Autodesk Inventor part; units mm, degrees
(part 2 of 3)
sketch "Эскиз3" plane through (0, 10, 0) normal (0, 1, 0) x (1, 0, 0)
  line L0 (-500, 500) -> (-500, -500) projected
  line L1 (-500, -500) -> (500, -500) projected
  line L2 (500, -500) -> (500, 500) projected
  line L3 (500, 500) -> (-500, 500) projected
  line L4 (-97.5, 500) -> (-102.5, 500) projected
  line L5 (-102.5, 500) -> (-102.5, 402.5) projected
  line L6 (-102.5, 402.5) -> (-197.5, 402.5) projected
  line L7 (-197.5, 402.5) -> (-197.5, 500) projected
  line L8 (-197.5, 500) -> (-202.5, 500) projected
  line L9 (-202.5, 500) -> (-202.5, 402.5) projected
  line L10 (-202.5, 402.5) -> (-297.5, 402.5) projected
  line L11 (-297.5, 402.5) -> (-297.5, 500) projected
  line L12 (-297.5, 500) -> (-302.5, 500) projected
  line L13 (-302.5, 500) -> (-302.5, 402.5) projected
  line L14 (-302.5, 402.5) -> (-397.5, 402.5) projected
  line L15 (-397.5, 402.5) -> (-397.5, 500) projected
  line L16 (-397.5, 500) -> (-402.5, 500) projected
  line L17 (-402.5, 500) -> (-402.5, 402.5) projected
  line L18 (-402.5, 402.5) -> (-500, 402.5) projected
  line L19 (-500, 402.5) -> (-500, 397.5) projected
  line L20 (-500, 397.5) -> (-402.5, 397.5) projected
  line L21 (-402.5, 397.5) -> (-402.5, 302.5) projected
  line L22 (-402.5, 302.5) -> (-500, 302.5) projected
  line L23 (-500, 302.5) -> (-500, 297.5) projected
  line L24 (-500, 297.5) -> (-402.5, 297.5) projected
  line L25 (-402.5, 297.5) -> (-402.5, 202.5) projected
  line L26 (-402.5, 202.5) -> (-500, 202.5) projected
  line L27 (-500, 202.5) -> (-500, 197.5) projected
  line L28 (-500, 197.5) -> (-402.5, 197.5) projected
  line L29 (-402.5, 197.5) -> (-402.5, 102.5) projected
  line L30 (-402.5, 102.5) -> (-500, 102.5) projected
  line L31 (-500, 102.5) -> (-500, 97.5) projected
  line L32 (-500, 97.5) -> (-402.5, 97.5) projected
  line L33 (-402.5, 97.5) -> (-402.5, 2.5) projected
  line L34 (-402.5, 2.5) -> (-500, 2.5) projected
  line L35 (-500, 2.5) -> (-500, -2.5) projected
  line L36 (-500, -2.5) -> (-402.5, -2.5) projected
  line L37 (-402.5, -2.5) -> (-402.5, -97.5) projected
  line L38 (-402.5, -97.5) -> (-500, -97.5) projected
  line L39 (-500, -97.5) -> (-500, -102.5) projected
  line L40 (-500, -102.5) -> (-402.5, -102.5) projected
  line L41 (-402.5, -102.5) -> (-402.5, -197.5) projected
  line L42 (-402.5, -197.5) -> (-500, -197.5) projected
  line L43 (-500, -197.5) -> (-500, -202.5) projected
  line L44 (-500, -202.5) -> (-402.5, -202.5) projected
  line L45 (-402.5, -202.5) -> (-402.5, -297.5) projected
  line L46 (-402.5, -297.5) -> (-500, -297.5) projected
  line L47 (-500, -297.5) -> (-500, -302.5) projected
  line L48 (-500, -302.5) -> (-402.5, -302.5) projected
  line L49 (-402.5, -302.5) -> (-402.5, -397.5) projected
  line L50 (-402.5, -397.5) -> (-500, -397.5) projected
  line L51 (-500, -397.5) -> (-500, -402.5) projected
  line L52 (-500, -402.5) -> (-402.5, -402.5) projected
  line L53 (-402.5, -402.5) -> (-402.5, -500) projected
  line L54 (-402.5, -500) -> (-397.5, -500) projected
  line L55 (-397.5, -500) -> (-397.5, -402.5) projected
  line L56 (-397.5, -402.5) -> (-302.5, -402.5) projected
  line L57 (-302.5, -402.5) -> (-302.5, -500) projected
  line L58 (-302.5, -500) -> (-297.5, -500) projected
  line L59 (-297.5, -500) -> (-297.5, -402.5) projected
  line L60 (-297.5, -402.5) -> (-202.5, -402.5) projected
  line L61 (-202.5, -402.5) -> (-202.5, -500) projected
  line L62 (-202.5, -500) -> (-197.5, -500) projected
  line L63 (-197.5, -500) -> (-197.5, -402.5) projected
  line L64 (-197.5, -402.5) -> (-102.5, -402.5) projected
  line L65 (-102.5, -402.5) -> (-102.5, -500) projected
  line L66 (-102.5, -500) -> (-97.5, -500) projected
  line L67 (-97.5, -500) -> (-97.5, -402.5) projected
  line L68 (-97.5, -402.5) -> (-2.5, -402.5) projected
  line L69 (-2.5, -402.5) -> (-2.5, -500) projected
  line L70 (-2.5, -500) -> (2.5, -500) projected
  line L71 (2.5, -500) -> (2.5, -402.5) projected
  line L72 (2.5, -402.5) -> (97.5, -402.5) projected
  line L73 (97.5, -402.5) -> (97.5, -500) projected
  line L74 (97.5, -500) -> (102.5, -500) projected
  line L75 (102.5, -500) -> (102.5, -402.5) projected
  line L76 (102.5, -402.5) -> (197.5, -402.5) projected
  line L77 (197.5, -402.5) -> (197.5, -500) projected
  line L78 (197.5, -500) -> (202.5, -500) projected
  line L79 (202.5, -500) -> (202.5, -402.5) projected
  line L80 (202.5, -402.5) -> (297.5, -402.5) projected
  line L81 (297.5, -402.5) -> (297.5, -500) projected
  line L82 (297.5, -500) -> (302.5, -500) projected
  line L83 (302.5, -500) -> (302.5, -402.5) projected
  line L84 (302.5, -402.5) -> (397.5, -402.5) projected
  line L85 (397.5, -402.5) -> (397.5, -500) projected
  line L86 (397.5, -500) -> (402.5, -500) projected
  line L87 (402.5, -500) -> (402.5, -402.5) projected
  line L88 (402.5, -402.5) -> (500, -402.5) projected
  line L89 (500, -402.5) -> (500, -397.5) projected
  line L90 (500, -397.5) -> (402.5, -397.5) projected
  line L91 (402.5, -397.5) -> (402.5, -302.5) projected
  line L92 (402.5, -302.5) -> (500, -302.5) projected
  line L93 (500, -302.5) -> (500, -297.5) projected
  line L94 (500, -297.5) -> (402.5, -297.5) projected
  line L95 (402.5, -297.5) -> (402.5, -202.5) projected
  line L96 (402.5, -202.5) -> (500, -202.5) projected
  line L97 (500, -202.5) -> (500, -197.5) projected
  line L98 (500, -197.5) -> (402.5, -197.5) projected
  line L99 (402.5, -197.5) -> (402.5, -102.5) projected
  line L100 (402.5, -102.5) -> (500, -102.5) projected
  line L101 (500, -102.5) -> (500, -97.5) projected
  line L102 (500, -97.5) -> (402.5, -97.5) projected
  line L103 (402.5, -97.5) -> (402.5, -2.5) projected
  line L104 (402.5, -2.5) -> (500, -2.5) projected
  line L105 (500, -2.5) -> (500, 2.5) projected
  line L106 (500, 2.5) -> (402.5, 2.5) projected
  line L107 (402.5, 2.5) -> (402.5, 97.5) projected
  line L108 (402.5, 97.5) -> (500, 97.5) projected
  line L109 (500, 97.5) -> (500, 102.5) projected
  line L110 (500, 102.5) -> (402.5, 102.5) projected
  line L111 (402.5, 102.5) -> (402.5, 197.5) projected
  line L112 (402.5, 197.5) -> (500, 197.5) projected
  line L113 (500, 197.5) -> (500, 202.5) projected
  line L114 (500, 202.5) -> (402.5, 202.5) projected
  line L115 (402.5, 202.5) -> (402.5, 297.5) projected
  line L116 (402.5, 297.5) -> (500, 297.5) projected
  line L117 (500, 297.5) -> (500, 302.5) projected
  line L118 (500, 302.5) -> (402.5, 302.5) projected
  line L119 (402.5, 302.5) -> (402.5, 397.5) projected
  line L120 (402.5, 397.5) -> (500, 397.5) projected
  line L121 (500, 397.5) -> (500, 402.5) projected
  line L122 (500, 402.5) -> (402.5, 402.5) projected
  line L123 (402.5, 402.5) -> (402.5, 500) projected
  line L124 (402.5, 500) -> (397.5, 500) projected
  line L125 (397.5, 500) -> (397.5, 402.5) projected
  line L126 (397.5, 402.5) -> (302.5, 402.5) projected
  line L127 (302.5, 402.5) -> (302.5, 500) projected
  line L128 (302.5, 500) -> (297.5, 500) projected
  line L129 (297.5, 500) -> (297.5, 402.5) projected
  line L130 (297.5, 402.5) -> (202.5, 402.5) projected
  line L131 (202.5, 402.5) -> (202.5, 500) projected
  line L132 (202.5, 500) -> (197.5, 500) projected
  line L133 (197.5, 500) -> (197.5, 402.5) projected
  line L134 (197.5, 402.5) -> (102.5, 402.5) projected
  line L135 (102.5, 402.5) -> (102.5, 500) projected
  line L136 (102.5, 500) -> (97.5, 500) projected
  line L137 (97.5, 500) -> (97.5, 402.5) projected
  line L138 (97.5, 402.5) -> (2.5, 402.5) projected
  line L139 (2.5, 402.5) -> (2.5, 500) projected
  line L140 (2.5, 500) -> (-2.5, 500) projected
  line L141 (-2.5, 500) -> (-2.5, 402.5) projected
  line L142 (-2.5, 402.5) -> (-97.5, 402.5) projected
  line L143 (-97.5, 402.5) -> (-97.5, 500) projected
  line L144 (197.5, -302.5) -> (197.5, -397.5) projected
  line L145 (197.5, -397.5) -> (102.5, -397.5) projected
  line L146 (102.5, -397.5) -> (102.5, -302.5) projected
  line L147 (102.5, -302.5) -> (197.5, -302.5) projected
  line L148 (197.5, -297.5) -> (102.5, -297.5) projected
  line L149 (102.5, -297.5) -> (102.5, -202.5) projected
  line L150 (102.5, -202.5) -> (197.5, -202.5) projected
  line L151 (197.5, -202.5) -> (197.5, -297.5) projected
  line L152 (97.5, -102.5) -> (97.5, -197.5) projected
  line L153 (97.5, -197.5) -> (2.5, -197.5) projected
  line L154 (2.5, -197.5) -> (2.5, -102.5) projected
  line L155 (2.5, -102.5) -> (97.5, -102.5) projected
  line L156 (97.5, -97.5) -> (2.5, -97.5) projected
  line L157 (2.5, -97.5) -> (2.5, -2.5) projected
  line L158 (2.5, -2.5) -> (97.5, -2.5) projected
  line L159 (97.5, -2.5) -> (97.5, -97.5) projected
  line L160 (-2.5, 97.5) -> (-2.5, 2.5) projected
  line L161 (-2.5, 2.5) -> (-97.5, 2.5) projected
  line L162 (-97.5, 2.5) -> (-97.5, 97.5) projected
  line L163 (-97.5, 97.5) -> (-2.5, 97.5) projected
  line L164 (-2.5, 102.5) -> (-97.5, 102.5) projected
  line L165 (-97.5, 102.5) -> (-97.5, 197.5) projected
  line L166 (-97.5, 197.5) -> (-2.5, 197.5) projected
  line L167 (-2.5, 197.5) -> (-2.5, 102.5) projected
  line L168 (-97.5, 397.5) -> (-2.5, 397.5) projected
  line L169 (-2.5, 397.5) -> (-2.5, 302.5) projected
  line L170 (-2.5, 302.5) -> (-97.5, 302.5) projected
  line L171 (-97.5, 302.5) -> (-97.5, 397.5) projected
  line L172 (-97.5, 297.5) -> (-2.5, 297.5) projected
  line L173 (-2.5, 297.5) -> (-2.5, 202.5) projected
  line L174 (-2.5, 202.5) -> (-97.5, 202.5) projected
  line L175 (-97.5, 202.5) -> (-97.5, 297.5) projected
  line L176 (-102.5, -302.5) -> (-102.5, -397.5) projected
  line L177 (-102.5, -397.5) -> (-197.5, -397.5) projected
  line L178 (-197.5, -397.5) -> (-197.5, -302.5) projected
  line L179 (-197.5, -302.5) -> (-102.5, -302.5) projected
  line L180 (-102.5, -202.5) -> (-102.5, -297.5) projected
  line L181 (-102.5, -297.5) -> (-197.5, -297.5) projected
  line L182 (-197.5, -297.5) -> (-197.5, -202.5) projected
  line L183 (-197.5, -202.5) -> (-102.5, -202.5) projected
  line L184 (-102.5, -102.5) -> (-102.5, -197.5) projected
  line L185 (-102.5, -197.5) -> (-197.5, -197.5) projected
  line L186 (-197.5, -197.5) -> (-197.5, -102.5) projected
  line L187 (-197.5, -102.5) -> (-102.5, -102.5) projected
  line L188 (-102.5, -2.5) -> (-102.5, -97.5) projected
  line L189 (-102.5, -97.5) -> (-197.5, -97.5) projected
  line L190 (-197.5, -97.5) -> (-197.5, -2.5) projected
  line L191 (-197.5, -2.5) -> (-102.5, -2.5) projected
  line L192 (-102.5, 97.5) -> (-102.5, 2.5) projected
  line L193 (-102.5, 2.5) -> (-197.5, 2.5) projected
  line L194 (-197.5, 2.5) -> (-197.5, 97.5) projected
  line L195 (-197.5, 97.5) -> (-102.5, 97.5) projected
  line L196 (-102.5, 197.5) -> (-102.5, 102.5) projected
  line L197 (-102.5, 102.5) -> (-197.5, 102.5) projected
  line L198 (-197.5, 102.5) -> (-197.5, 197.5) projected
  line L199 (-197.5, 197.5) -> (-102.5, 197.5) projected
  line L200 (-102.5, 297.5) -> (-102.5, 202.5) projected
  line L201 (-102.5, 202.5) -> (-197.5, 202.5) projected
  line L202 (-197.5, 202.5) -> (-197.5, 297.5) projected
  line L203 (-197.5, 297.5) -> (-102.5, 297.5) projected
  line L204 (-102.5, 397.5) -> (-102.5, 302.5) projected
  line L205 (-102.5, 302.5) -> (-197.5, 302.5) projected
  line L206 (-197.5, 302.5) -> (-197.5, 397.5) projected
  line L207 (-197.5, 397.5) -> (-102.5, 397.5) projected
  line L208 (-97.5, -302.5) -> (-2.5, -302.5) projected
  line L209 (-2.5, -302.5) -> (-2.5, -397.5) projected
  line L210 (-2.5, -397.5) -> (-97.5, -397.5) projected
  line L211 (-97.5, -397.5) -> (-97.5, -302.5) projected
  line L212 (-202.5, -302.5) -> (-202.5, -397.5) projected
  line L213 (-202.5, -397.5) -> (-297.5, -397.5) projected
  line L214 (-297.5, -397.5) -> (-297.5, -302.5) projected
  line L215 (-297.5, -302.5) -> (-202.5, -302.5) projected
  line L216 (-202.5, -297.5) -> (-297.5, -297.5) projected
  line L217 (-297.5, -297.5) -> (-297.5, -202.5) projected
  line L218 (-297.5, -202.5) -> (-202.5, -202.5) projected
  line L219 (-202.5, -202.5) -> (-202.5, -297.5) projected
  line L220 (2.5, 102.5) -> (2.5, 197.5) projected
  line L221 (2.5, 197.5) -> (97.5, 197.5) projected
  line L222 (97.5, 197.5) -> (97.5, 102.5) projected
  line L223 (97.5, 102.5) -> (2.5, 102.5) projected
  line L224 (-297.5, 397.5) -> (-202.5, 397.5) projected
  line L225 (-202.5, 397.5) -> (-202.5, 302.5) projected
  line L226 (-202.5, 302.5) -> (-297.5, 302.5) projected
  line L227 (-297.5, 302.5) -> (-297.5, 397.5) projected
  line L228 (-297.5, 297.5) -> (-202.5, 297.5) projected
  line L229 (-202.5, 297.5) -> (-202.5, 202.5) projected
  line L230 (-202.5, 202.5) -> (-297.5, 202.5) projected
  line L231 (-297.5, 202.5) -> (-297.5, 297.5) projected
  line L232 (-297.5, 197.5) -> (-202.5, 197.5) projected
  line L233 (-202.5, 197.5) -> (-202.5, 102.5) projected
  line L234 (-202.5, 102.5) -> (-297.5, 102.5) projected
  line L235 (-297.5, 102.5) -> (-297.5, 197.5) projected
  line L236 (-297.5, 97.5) -> (-202.5, 97.5) projected
  line L237 (-202.5, 97.5) -> (-202.5, 2.5) projected
  line L238 (-202.5, 2.5) -> (-297.5, 2.5) projected
  line L239 (-297.5, 2.5) -> (-297.5, 97.5) projected
  line L240 (-297.5, -2.5) -> (-202.5, -2.5) projected
  line L241 (-202.5, -2.5) -> (-202.5, -97.5) projected
  line L242 (-202.5, -97.5) -> (-297.5, -97.5) projected
  line L243 (-297.5, -97.5) -> (-297.5, -2.5) projected
  line L244 (-297.5, -102.5) -> (-202.5, -102.5) projected
  line L245 (-202.5, -102.5) -> (-202.5, -197.5) projected
  line L246 (-202.5, -197.5) -> (-297.5, -197.5) projected
  line L247 (-297.5, -197.5) -> (-297.5, -102.5) projected
  line L248 (-302.5, -302.5) -> (-302.5, -397.5) projected
  line L249 (-302.5, -397.5) -> (-397.5, -397.5) projected
  line L250 (-397.5, -397.5) -> (-397.5, -302.5) projected
  line L251 (-397.5, -302.5) -> (-302.5, -302.5) projected
  line L252 (-302.5, -202.5) -> (-302.5, -297.5) projected
  line L253 (-302.5, -297.5) -> (-397.5, -297.5) projected
  line L254 (-397.5, -297.5) -> (-397.5, -202.5) projected
  line L255 (-397.5, -202.5) -> (-302.5, -202.5) projected
  line L256 (-302.5, -102.5) -> (-302.5, -197.5) projected
  line L257 (-302.5, -197.5) -> (-397.5, -197.5) projected
  line L258 (-397.5, -197.5) -> (-397.5, -102.5) projected
  line L259 (-397.5, -102.5) -> (-302.5, -102.5) projected
  line L260 (-302.5, -2.5) -> (-302.5, -97.5) projected
  line L261 (-302.5, -97.5) -> (-397.5, -97.5) projected
  line L262 (-397.5, -97.5) -> (-397.5, -2.5) projected
  line L263 (-397.5, -2.5) -> (-302.5, -2.5) projected
  line L264 (-302.5, 97.5) -> (-302.5, 2.5) projected
  line L265 (-302.5, 2.5) -> (-397.5, 2.5) projected
  line L266 (-397.5, 2.5) -> (-397.5, 97.5) projected
  line L267 (-397.5, 97.5) -> (-302.5, 97.5) projected
  line L268 (-302.5, 197.5) -> (-302.5, 102.5) projected
  line L269 (-302.5, 102.5) -> (-397.5, 102.5) projected
  line L270 (-397.5, 102.5) -> (-397.5, 197.5) projected
  line L271 (-397.5, 197.5) -> (-302.5, 197.5) projected
  line L272 (-302.5, 297.5) -> (-302.5, 202.5) projected
  line L273 (-302.5, 202.5) -> (-397.5, 202.5) projected
  line L274 (-397.5, 202.5) -> (-397.5, 297.5) projected
  line L275 (-397.5, 297.5) -> (-302.5, 297.5) projected
  line L276 (-302.5, 397.5) -> (-302.5, 302.5) projected
  line L277 (-302.5, 302.5) -> (-397.5, 302.5) projected
  line L278 (-397.5, 302.5) -> (-397.5, 397.5) projected
  line L279 (-397.5, 397.5) -> (-302.5, 397.5) projected
  line L280 (-97.5, -102.5) -> (-2.5, -102.5) projected
  line L281 (-2.5, -102.5) -> (-2.5, -197.5) projected
  line L282 (-2.5, -197.5) -> (-97.5, -197.5) projected
  line L283 (-97.5, -197.5) -> (-97.5, -102.5) projected
  line L284 (-97.5, -2.5) -> (-2.5, -2.5) projected
  line L285 (-2.5, -2.5) -> (-2.5, -97.5) projected
  line L286 (-2.5, -97.5) -> (-97.5, -97.5) projected
  line L287 (-97.5, -97.5) -> (-97.5, -2.5) projected
  line L288 (2.5, 97.5) -> (97.5, 97.5) projected
  line L289 (97.5, 97.5) -> (97.5, 2.5) projected
  line L290 (97.5, 2.5) -> (2.5, 2.5) projected
  line L291 (2.5, 2.5) -> (2.5, 97.5) projected
  line L292 (202.5, -297.5) -> (202.5, -202.5) projected
  line L293 (202.5, -202.5) -> (297.5, -202.5) projected
  line L294 (297.5, -202.5) -> (297.5, -297.5) projected
  line L295 (297.5, -297.5) -> (202.5, -297.5) projected
  line L296 (102.5, -102.5) -> (197.5, -102.5) projected
  line L297 (197.5, -102.5) -> (197.5, -197.5) projected
  line L298 (197.5, -197.5) -> (102.5, -197.5) projected
  line L299 (102.5, -197.5) -> (102.5, -102.5) projected
  line L300 (202.5, -302.5) -> (297.5, -302.5) projected
  line L301 (297.5, -302.5) -> (297.5, -397.5) projected
  line L302 (297.5, -397.5) -> (202.5, -397.5) projected
  line L303 (202.5, -397.5) -> (202.5, -302.5) projected
  line L304 (202.5, -97.5) -> (202.5, -2.5) projected
  line L305 (202.5, -2.5) -> (297.5, -2.5) projected
  line L306 (297.5, -2.5) -> (297.5, -97.5) projected
  line L307 (297.5, -97.5) -> (202.5, -97.5) projected
  line L308 (197.5, 2.5) -> (102.5, 2.5) projected
  line L309 (102.5, 2.5) -> (102.5, 97.5) projected
  line L310 (102.5, 97.5) -> (197.5, 97.5) projected
  line L311 (197.5, 97.5) -> (197.5, 2.5) projected
  line L312 (202.5, 102.5) -> (202.5, 197.5) projected
  line L313 (202.5, 197.5) -> (297.5, 197.5) projected
  line L314 (297.5, 197.5) -> (297.5, 102.5) projected
  line L315 (297.5, 102.5) -> (202.5, 102.5) projected
  line L316 (197.5, 202.5) -> (102.5, 202.5) projected
  line L317 (102.5, 202.5) -> (102.5, 297.5) projected
  line L318 (102.5, 297.5) -> (197.5, 297.5) projected
  line L319 (197.5, 297.5) -> (197.5, 202.5) projected
  line L320 (202.5, 302.5) -> (202.5, 397.5) projected
  line L321 (202.5, 397.5) -> (297.5, 397.5) projected
  line L322 (297.5, 397.5) -> (297.5, 302.5) projected
  line L323 (297.5, 302.5) -> (202.5, 302.5) projected
  line L324 (97.5, -202.5) -> (97.5, -297.5) projected
  line L325 (97.5, -297.5) -> (2.5, -297.5) projected
  line L326 (2.5, -297.5) -> (2.5, -202.5) projected
  line L327 (2.5, -202.5) -> (97.5, -202.5) projected
  line L328 (97.5, -302.5) -> (97.5, -397.5) projected
  line L329 (97.5, -397.5) -> (2.5, -397.5) projected
  line L330 (2.5, -397.5) -> (2.5, -302.5) projected
  line L331 (2.5, -302.5) -> (97.5, -302.5) projected
  line L332 (302.5, -302.5) -> (397.5, -302.5) projected
  line L333 (397.5, -302.5) -> (397.5, -397.5) projected
  line L334 (397.5, -397.5) -> (302.5, -397.5) projected
  line L335 (302.5, -397.5) -> (302.5, -302.5) projected
  line L336 (302.5, -202.5) -> (397.5, -202.5) projected
  line L337 (397.5, -202.5) -> (397.5, -297.5) projected
  line L338 (397.5, -297.5) -> (302.5, -297.5) projected
  line L339 (302.5, -297.5) -> (302.5, -202.5) projected
  line L340 (302.5, -102.5) -> (397.5, -102.5) projected
  line L341 (397.5, -102.5) -> (397.5, -197.5) projected
  line L342 (397.5, -197.5) -> (302.5, -197.5) projected
  line L343 (302.5, -197.5) -> (302.5, -102.5) projected
  line L344 (302.5, -2.5) -> (397.5, -2.5) projected
  line L345 (397.5, -2.5) -> (397.5, -97.5) projected
  line L346 (397.5, -97.5) -> (302.5, -97.5) projected
  line L347 (302.5, -97.5) -> (302.5, -2.5) projected
  line L348 (302.5, 97.5) -> (397.5, 97.5) projected
  line L349 (397.5, 97.5) -> (397.5, 2.5) projected
  line L350 (397.5, 2.5) -> (302.5, 2.5) projected
  line L351 (302.5, 2.5) -> (302.5, 97.5) projected
  line L352 (302.5, 197.5) -> (397.5, 197.5) projected
  line L353 (397.5, 197.5) -> (397.5, 102.5) projected
  line L354 (397.5, 102.5) -> (302.5, 102.5) projected
  line L355 (302.5, 102.5) -> (302.5, 197.5) projected
  line L356 (302.5, 297.5) -> (397.5, 297.5) projected
  line L357 (397.5, 297.5) -> (397.5, 202.5) projected
  line L358 (397.5, 202.5) -> (302.5, 202.5) projected
  line L359 (302.5, 202.5) -> (302.5, 297.5) projected
  line L360 (302.5, 397.5) -> (397.5, 397.5) projected
  line L361 (397.5, 397.5) -> (397.5, 302.5) projected
  line L362 (397.5, 302.5) -> (302.5, 302.5) projected
  line L363 (302.5, 302.5) -> (302.5, 397.5) projected
  line L364 (97.5, 202.5) -> (2.5, 202.5) projected
  line L365 (2.5, 202.5) -> (2.5, 297.5) projected
  line L366 (2.5, 297.5) -> (97.5, 297.5) projected
  line L367 (97.5, 297.5) -> (97.5, 202.5) projected
  line L368 (97.5, 302.5) -> (2.5, 302.5) projected
  line L369 (2.5, 302.5) -> (2.5, 397.5) projected
  line L370 (2.5, 397.5) -> (97.5, 397.5) projected
  line L371 (97.5, 397.5) -> (97.5, 302.5) projected
  line L372 (197.5, 302.5) -> (102.5, 302.5) projected
  line L373 (102.5, 302.5) -> (102.5, 397.5) projected
  line L374 (102.5, 397.5) -> (197.5, 397.5) projected
  line L375 (197.5, 397.5) -> (197.5, 302.5) projected
  line L376 (202.5, 202.5) -> (202.5, 297.5) projected
  line L377 (202.5, 297.5) -> (297.5, 297.5) projected
  line L378 (297.5, 297.5) -> (297.5, 202.5) projected
  line L379 (297.5, 202.5) -> (202.5, 202.5) projected
  line L380 (197.5, 102.5) -> (102.5, 102.5) projected
  line L381 (102.5, 102.5) -> (102.5, 197.5) projected
  line L382 (102.5, 197.5) -> (197.5, 197.5) projected
  line L383 (197.5, 197.5) -> (197.5, 102.5) projected
  line L384 (202.5, 2.5) -> (202.5, 97.5) projected
  line L385 (202.5, 97.5) -> (297.5, 97.5) projected
  line L386 (297.5, 97.5) -> (297.5, 2.5) projected
  line L387 (297.5, 2.5) -> (202.5, 2.5) projected
  line L388 (102.5, -97.5) -> (102.5, -2.5) projected
  line L389 (102.5, -2.5) -> (197.5, -2.5) projected
  line L390 (197.5, -2.5) -> (197.5, -97.5) projected
  line L391 (197.5, -97.5) -> (102.5, -97.5) projected
  line L392 (202.5, -197.5) -> (202.5, -102.5) projected
  line L393 (202.5, -102.5) -> (297.5, -102.5) projected
  line L394 (297.5, -102.5) -> (297.5, -197.5) projected
  line L395 (297.5, -197.5) -> (202.5, -197.5) projected
  line L396 (-97.5, -202.5) -> (-2.5, -202.5) projected
  line L397 (-2.5, -202.5) -> (-2.5, -297.5) projected
  line L398 (-2.5, -297.5) -> (-97.5, -297.5) projected
  line L399 (-97.5, -297.5) -> (-97.5, -202.5) projected
  point P0 (0, 0)
extrude "Выдавливание3" add sketch "Эскиз3" along normal blind 0.1 separate body contours L3 L141 L142 L143 | L3 L2 L122 L123 | L2 L102 L103 L104
sketch "Эскиз4" plane through (0, 10.1, 0) normal (0, 1, 0) x (1, 0, 0)
  line L0 (402.5, -97.5) -> (500, -97.5) projected
  line L1 (500, -97.5) -> (500, -2.5) projected
  line L2 (500, -2.5) -> (402.5, -2.5) projected
  line L3 (402.5, -2.5) -> (402.5, -97.5) projected
  circle A0 centre (451.25, -50) radius 30
  line L4 (-2.5, 402.5) -> (-2.5, 500) projected
  line L5 (-2.5, 500) -> (-97.5, 500) projected
  line L6 (-97.5, 500) -> (-97.5, 402.5) projected
  line L7 (-97.5, 402.5) -> (-2.5, 402.5) projected
  circle A1 centre (-50, 451.25) radius 30
  circle A2 centre (451.25, 451.25) radius 30
  point P0 (0, 0)
  dimension "d21" = 60
  dimension "d22" = 60
  dimension "d23" = 60
  constraints: 3 centre point
  measures "d21" diameter of A0
  measures "d22" diameter of A1
  measures "d23" diameter of A2
extrude "Выдавливание4" add sketch "Эскиз4" along normal blind 0.1 separate body contours A0
sketch "Эскиз5" plane through (0, 10.1, 0) normal (0, 1, 0) x (1, 0, 0)
  line L0 (-2.5, 402.5) -> (-2.5, 500) projected
  line L1 (-2.5, 500) -> (-97.5, 500) projected
  line L2 (-97.5, 500) -> (-97.5, 402.5) projected
  line L3 (-97.5, 402.5) -> (-2.5, 402.5) projected
  circle A0 centre (-50, 451.25) radius 30
  point P0 (0, 0)
  dimension "d26" = 60
  constraints: 1 centre point
  measures "d26" diameter of A0
extrude "Выдавливание5" add sketch "Эскиз5" along normal blind 0.1 separate body contours A0
sketch "Эскиз6" plane through (0, 10.1, 0) normal (0, 1, 0) x (1, 0, 0)
  line L0 (402.5, 402.5) -> (500, 402.5) projected
  line L1 (500, 402.5) -> (500, 500) projected
  line L2 (500, 500) -> (402.5, 500) projected
  line L3 (402.5, 500) -> (402.5, 402.5) projected
  circle A0 centre (451.25, 451.25) radius 30
  point P0 (0, 0)
  dimension "d29" = 60
  constraints: 1 centre point
  measures "d29" diameter of A0
extrude "Выдавливание6" add sketch "Эскиз6" along normal blind 0.1 separate body contours A0
sketch "Эскиз7" plane through (0, 10, 0) normal (0, 1, 0) x (1, 0, 0)
  line L0 (403.4355, 616.1633) -> (-59.882, 616.1633) construction
  line L1 (-59.882, 616.1633) -> (-59.882, 831.1669) construction
  line L2 (-59.882, 831.1669) -> (403.4355, 831.1669) construction
  line L3 (403.4355, 831.1669) -> (403.4355, 616.1633) construction
  line L4 (727.2768, 390.1714) -> (727.2768, -106.4566) construction
  line L5 (727.2768, -106.4566) -> (536.499, -106.4566) construction
  line L6 (536.499, -106.4566) -> (536.499, 390.1714) construction
  line L7 (536.499, 390.1714) -> (727.2768, 390.1714) construction
  line L8 (478.0191, 533.7037) -> (-758.7596, 533.7037) construction
  line L9 (-758.7596, 533.7037) -> (-758.7596, 958.9176) construction
  line L10 (-758.7596, 958.9176) -> (478.0191, 958.9176) construction
  line L11 (478.0191, 958.9176) -> (478.0191, 533.7037) construction
  line L12 (592.7727, 476.9268) -> (592.7727, -759.8518) construction
  line L13 (592.7727, -759.8518) -> (167.5588, -759.8518) construction
  line L14 (167.5588, -759.8518) -> (167.5588, 476.9268) construction
  line L15 (167.5588, 476.9268) -> (592.7727, 476.9268) construction
  spline S0 degree 2 poles (322.5603, 629.6965) (316.8877, 636.3416) (310.5668, 655.7905) (310.5668, 668.2703) knots 0 0 0 1 2 2 2
  spline S1 degree 2 poles (310.5668, 668.2703) (310.5668, 680.4259) (316.7256, 700.1179) (322.5603, 706.763) knots 0 0 0 1 2 2 2
  spline S2 degree 2 poles (322.5603, 706.763) (328.7191, 713.7322) (345.0076, 720.3772) (354.8131, 720.3772) knots 0 0 0 1 2 2 2
  spline S3 degree 2 poles (354.8131, 720.3772) (364.9428, 720.3772) (381.1503, 713.4891) (387.066, 706.763) knots 0 0 0 1 2 2 2
  spline S4 degree 2 poles (387.066, 706.763) (392.8196, 700.1179) (398.9785, 680.5879) (398.9785, 668.2703) knots 0 0 0 1 2 2 2
  spline S5 degree 2 poles (398.9785, 668.2703) (398.9785, 655.7095) (392.7386, 636.5847) (386.9849, 629.6965) knots 0 0 0 1 2 2 2
  spline S6 degree 2 poles (386.9849, 629.6965) (381.1503, 623.0515) (364.8618, 616.1633) (354.8131, 616.1633) knots 0 0 0 1 2 2 2
  spline S7 degree 2 poles (354.8131, 616.1633) (344.6024, 616.1633) (328.2329, 623.2946) (322.5603, 629.6965) knots 0 0 0 1 2 2 2
  spline S8 degree 2 poles (324.4242, 668.2703) (324.4242, 658.3837) (328.7191, 643.0677) (332.6089, 638.0434) knots 0 0 0 1 2 2 2
  spline S9 degree 2 poles (332.6089, 638.0434) (336.5798, 632.857) (347.7629, 627.6706) (354.7321, 627.6706) knots 0 0 0 1 2 2 2
  spline S10 degree 2 poles (354.7321, 627.6706) (361.9444, 627.6706) (372.8034, 632.6949) (376.9363, 638.0434) knots 0 0 0 1 2 2 2
  spline S11 degree 2 poles (376.9363, 638.0434) (380.9071, 643.1487) (385.1211, 658.5458) (385.1211, 668.2703) knots 0 0 0 1 2 2 2
  spline S12 degree 2 poles (385.1211, 668.2703) (385.1211, 687.9623) (368.5895, 708.87) (354.7321, 708.87) knots 0 0 0 1 2 2 2
  spline S13 degree 2 poles (354.7321, 708.87) (340.8747, 708.87) (324.4242, 687.9623) (324.4242, 668.2703) knots 0 0 0 1 2 2 2
  spline S14 degree 2 poles (267.1308, 719.9721) (274.9104, 719.9721) (287.7953, 715.1909) (292.4144, 710.3286) knots 0 0 0 1 2 2 2
  spline S15 degree 2 poles (292.4144, 710.3286) (297.0336, 705.5474) (302.1389, 690.7986) (302.1389, 680.9121) knots 0 0 0 1 2 2 2
  spline S16 degree 2 poles (302.1389, 680.9121) (302.1389, 671.0255) (296.8715, 656.6009) (292.4144, 651.7387) knots 0 0 0 1 2 2 2
  spline S17 degree 2 poles (292.4144, 651.7387) (287.9574, 646.7954) (274.7483, 641.528) (267.1308, 641.528) knots 0 0 0 1 2 2 2
  spline S18 degree 2 poles (267.1308, 641.528) (260.972, 641.528) (249.4647, 645.0126) (245.0076, 647.2816) knots 0 0 0 1 2 2 2
  line L16 (245.0076, 647.2816) -> (245.0076, 661.4631)
  line L17 (245.0076, 661.4631) -> (245.737, 661.4631)
  spline S19 degree 2 poles (245.737, 661.4631) (247.1146, 660.3286) (251.3285, 657.4113) (254.3269, 655.8716) knots 0 0 0 1 2 2 2
  spline S20 degree 2 poles (254.3269, 655.8716) (257.0011, 654.575) (264.1324, 652.549) (267.3739, 652.549) knots 0 0 0 1 2 2 2
  spline S21 degree 2 poles (267.3739, 652.549) (277.1794, 652.549) (289.0919, 667.3789) (289.0919, 680.9121) knots 0 0 0 1 2 2 2
  spline S22 degree 2 poles (289.0919, 680.9121) (289.0919, 694.1212) (277.5846, 708.951) (267.3739, 708.951) knots 0 0 0 1 2 2 2
  spline S23 degree 2 poles (267.3739, 708.951) (261.2151, 708.951) (250.0319, 703.8456) (245.737, 699.8748) knots 0 0 0 1 2 2 2
  line L18 (245.737, 699.8748) -> (245.0076, 699.8748)
  line L19 (245.0076, 699.8748) -> (245.0076, 714.0563)
  spline S24 degree 2 poles (245.0076, 714.0563) (246.8715, 714.9477) (252.5441, 717.4599) (254.8131, 718.0272) knots 0 0 0 1 2 2 2
  spline S25 degree 2 poles (254.8131, 718.0272) (258.0546, 718.9996) (263.16, 719.9721) (267.1308, 719.9721) knots 0 0 0 1 2 2 2
  spline S26 degree 2 poles (176.7742, 695.0126) (176.7742, 700.4421) (181.1503, 709.3562) (184.878, 712.1114) knots 0 0 0 1 2 2 2
  spline S27 degree 2 poles (184.878, 712.1114) (189.335, 715.434) (199.3836, 718.2703) (207.2443, 718.2703) knots 0 0 0 1 2 2 2
  line L20 (207.2443, 718.2703) -> (233.5003, 718.2703)
  line L21 (233.5003, 718.2703) -> (233.5003, 643.2298)
  line L22 (233.5003, 643.2298) -> (220.8585, 643.2298)
  line L23 (220.8585, 643.2298) -> (220.8585, 672.4842)
  line L24 (220.8585, 672.4842) -> (206.9201, 672.4842)
  spline S28 degree 2 poles (206.9201, 672.4842) (198.4922, 672.4842) (189.1729, 674.267) (184.5538, 677.6706) knots 0 0 0 1 2 2 2
  spline S29 degree 2 poles (184.5538, 677.6706) (180.664, 680.5069) (176.7742, 689.502) (176.7742, 695.0126) knots 0 0 0 1 2 2 2
  spline S30 degree 2 poles (189.8212, 695.2557) (189.8212, 691.8521) (192.1713, 686.6657) (194.8456, 685.045) knots 0 0 0 1 2 2 2
  spline S31 degree 2 poles (194.8456, 685.045) (197.6819, 683.3432) (204.8131, 682.6949) (211.4582, 682.6949) knots 0 0 0 1 2 2 2
  line L25 (211.4582, 682.6949) -> (220.8585, 682.6949)
  line L26 (220.8585, 682.6949) -> (220.8585, 708.2217)
  line L27 (220.8585, 708.2217) -> (211.7823, 708.2217)
  spline S32 degree 2 poles (211.7823, 708.2217) (205.0563, 708.2217) (197.6819, 707.0871) (195.0076, 705.4664) knots 0 0 0 1 2 2 2
  spline S33 degree 2 poles (195.0076, 705.4664) (192.3334, 703.6836) (189.8212, 698.9834) (189.8212, 695.2557) knots 0 0 0 1 2 2 2
  line L28 (51.6527, 718.2703) -> (66.8877, 718.2703)
  line L29 (66.8877, 718.2703) -> (91.1989, 678.3999)
  line L30 (91.1989, 678.3999) -> (115.9963, 718.2703)
  line L31 (115.9963, 718.2703) -> (130.3399, 718.2703)
  line L32 (130.3399, 718.2703) -> (98.4922, 668.1892)
  line L33 (98.4922, 668.1892) -> (129.3674, 618.2703)
  line L34 (129.3674, 618.2703) -> (114.1324, 618.2703)
  line L35 (114.1324, 618.2703) -> (90.3075, 657.4113)
  line L36 (90.3075, 657.4113) -> (65.9963, 618.2703)
  line L37 (65.9963, 618.2703) -> (51.6527, 618.2703)
  line L38 (51.6527, 618.2703) -> (82.9331, 667.5409)
  line L39 (82.9331, 667.5409) -> (51.6527, 718.2703)
  spline S34 degree 2 poles (713.7436, 309.2962) (707.0985, 303.6236) (687.6496, 297.3027) (675.1698, 297.3027) knots 0 0 0 1 2 2 2
  spline S35 degree 2 poles (675.1698, 297.3027) (663.0142, 297.3027) (643.3222, 303.4615) (636.6771, 309.2962) knots 0 0 0 1 2 2 2
  spline S36 degree 2 poles (636.6771, 309.2962) (629.7079, 315.455) (623.0629, 331.7435) (623.0629, 341.549) knots 0 0 0 1 2 2 2
  spline S37 degree 2 poles (623.0629, 341.549) (623.0629, 351.6787) (629.951, 367.8861) (636.6771, 373.8018) knots 0 0 0 1 2 2 2
  spline S38 degree 2 poles (636.6771, 373.8018) (643.3222, 379.5555) (662.8522, 385.7143) (675.1698, 385.7143) knots 0 0 0 1 2 2 2
  spline S39 degree 2 poles (675.1698, 385.7143) (687.7306, 385.7143) (706.8554, 379.4745) (713.7436, 373.7208) knots 0 0 0 1 2 2 2
  spline S40 degree 2 poles (713.7436, 373.7208) (720.3886, 367.8861) (727.2768, 351.5976) (727.2768, 341.549) knots 0 0 0 1 2 2 2
  spline S41 degree 2 poles (727.2768, 341.549) (727.2768, 331.3383) (720.1455, 314.9688) (713.7436, 309.2962) knots 0 0 0 1 2 2 2
  spline S42 degree 2 poles (675.1698, 311.16) (685.0564, 311.16) (700.3724, 315.455) (705.3967, 319.3448) knots 0 0 0 1 2 2 2
  spline S43 degree 2 poles (705.3967, 319.3448) (710.5831, 323.3156) (715.7695, 334.4988) (715.7695, 341.468) knots 0 0 0 1 2 2 2
  spline S44 degree 2 poles (715.7695, 341.468) (715.7695, 348.6803) (710.7452, 359.5393) (705.3967, 363.6722) knots 0 0 0 1 2 2 2
  spline S45 degree 2 poles (705.3967, 363.6722) (700.2914, 367.643) (684.8943, 371.857) (675.1698, 371.857) knots 0 0 0 1 2 2 2
  spline S46 degree 2 poles (675.1698, 371.857) (655.4778, 371.857) (634.5702, 355.3253) (634.5702, 341.468) knots 0 0 0 1 2 2 2
  spline S47 degree 2 poles (634.5702, 341.468) (634.5702, 327.6106) (655.4778, 311.16) (675.1698, 311.16) knots 0 0 0 1 2 2 2
  spline S48 degree 2 poles (623.4681, 253.8667) (623.4681, 261.6463) (628.2493, 274.5312) (633.1115, 279.1503) knots 0 0 0 1 2 2 2
  spline S49 degree 2 poles (633.1115, 279.1503) (637.8927, 283.7694) (652.6415, 288.8748) (662.528, 288.8748) knots 0 0 0 1 2 2 2
  spline S50 degree 2 poles (662.528, 288.8748) (672.4146, 288.8748) (686.8392, 283.6074) (691.7014, 279.1503) knots 0 0 0 1 2 2 2
  spline S51 degree 2 poles (691.7014, 279.1503) (696.6447, 274.6933) (701.9121, 261.4842) (701.9121, 253.8667) knots 0 0 0 1 2 2 2
  spline S52 degree 2 poles (701.9121, 253.8667) (701.9121, 247.7078) (698.4275, 236.2005) (696.1585, 231.7435) knots 0 0 0 1 2 2 2
  line L40 (696.1585, 231.7435) -> (681.977, 231.7435)
  line L41 (681.977, 231.7435) -> (681.977, 232.4728)
  spline S53 degree 2 poles (681.977, 232.4728) (683.1115, 233.8505) (686.0288, 238.0644) (687.5685, 241.0628) knots 0 0 0 1 2 2 2
  spline S54 degree 2 poles (687.5685, 241.0628) (688.8651, 243.737) (690.8911, 250.8683) (690.8911, 254.1098) knots 0 0 0 1 2 2 2
  spline S55 degree 2 poles (690.8911, 254.1098) (690.8911, 263.9153) (676.0612, 275.8278) (662.528, 275.8278) knots 0 0 0 1 2 2 2
  spline S56 degree 2 poles (662.528, 275.8278) (649.3189, 275.8278) (634.4891, 264.3205) (634.4891, 254.1098) knots 0 0 0 1 2 2 2
  spline S57 degree 2 poles (634.4891, 254.1098) (634.4891, 247.951) (639.5945, 236.7678) (643.5653, 232.4728) knots 0 0 0 1 2 2 2
  line L42 (643.5653, 232.4728) -> (643.5653, 231.7435)
  line L43 (643.5653, 231.7435) -> (629.3838, 231.7435)
  spline S58 degree 2 poles (629.3838, 231.7435) (628.4924, 233.6074) (625.9802, 239.28) (625.4129, 241.549) knots 0 0 0 1 2 2 2
  spline S59 degree 2 poles (625.4129, 241.549) (624.4405, 244.7905) (623.4681, 249.8958) (623.4681, 253.8667) knots 0 0 0 1 2 2 2
  spline S60 degree 2 poles (648.4275, 163.5101) (642.998, 163.5101) (634.0839, 167.8861) (631.3287, 171.6138) knots 0 0 0 1 2 2 2
  spline S61 degree 2 poles (631.3287, 171.6138) (628.0061, 176.0709) (625.1698, 186.1195) (625.1698, 193.9801) knots 0 0 0 1 2 2 2
  line L44 (625.1698, 193.9801) -> (625.1698, 220.2362)
  line L45 (625.1698, 220.2362) -> (700.2104, 220.2362)
  line L46 (700.2104, 220.2362) -> (700.2104, 207.5944)
  line L47 (700.2104, 207.5944) -> (670.9559, 207.5944)
  line L48 (670.9559, 207.5944) -> (670.9559, 193.656)
  spline S62 degree 2 poles (670.9559, 193.656) (670.9559, 185.2281) (669.1731, 175.9088) (665.7695, 171.2897) knots 0 0 0 1 2 2 2
  spline S63 degree 2 poles (665.7695, 171.2897) (662.9332, 167.3999) (653.9381, 163.5101) (648.4275, 163.5101) knots 0 0 0 1 2 2 2
  spline S64 degree 2 poles (648.1844, 176.5571) (651.588, 176.5571) (656.7744, 178.9072) (658.3951, 181.5814) knots 0 0 0 1 2 2 2
  spline S65 degree 2 poles (658.3951, 181.5814) (660.0969, 184.4177) (660.7452, 191.549) (660.7452, 198.1941) knots 0 0 0 1 2 2 2
  line L49 (660.7452, 198.1941) -> (660.7452, 207.5944)
  line L50 (660.7452, 207.5944) -> (635.2185, 207.5944)
  line L51 (635.2185, 207.5944) -> (635.2185, 198.5182)
  spline S66 degree 2 poles (635.2185, 198.5182) (635.2185, 191.7921) (636.353, 184.4177) (637.9737, 181.7435) knots 0 0 0 1 2 2 2
  spline S67 degree 2 poles (637.9737, 181.7435) (639.7565, 179.0693) (644.4567, 176.5571) (648.1844, 176.5571) knots 0 0 0 1 2 2 2
  line L52 (725.1698, 37.4971) -> (669.4162, 71.2897)
  line L53 (669.4162, 71.2897) -> (625.1698, 71.2897)
  line L54 (625.1698, 71.2897) -> (625.1698, 84.5798)
  line L55 (625.1698, 84.5798) -> (668.0386, 84.5798)
  line L56 (668.0386, 84.5798) -> (725.1698, 118.3723)
  line L57 (725.1698, 118.3723) -> (725.1698, 103.6236)
  line L58 (725.1698, 103.6236) -> (681.1666, 77.8537)
  line L59 (681.1666, 77.8537) -> (725.1698, 51.5976)
  line L60 (725.1698, 51.5976) -> (725.1698, 37.4971)
  spline S68 degree 2 poles (565.5928, 440.7712) (551.6025, 440.7712) (538.4971, 448.9041) (538.4971, 457.3741) knots 0 0 0 1 2 2 2
  spline S69 degree 2 poles (538.4971, 457.3741) (538.4971, 465.9706) (551.8553, 474.0192) (565.5506, 474.0192) knots 0 0 0 1 2 2 2
  spline S70 degree 2 poles (565.5506, 474.0192) (579.6252, 474.0192) (592.6463, 465.8863) (592.6463, 457.3741) knots 0 0 0 1 2 2 2
  spline S71 degree 2 poles (592.6463, 457.3741) (592.6463, 448.8198) (579.1617, 440.7712) (565.5928, 440.7712) knots 0 0 0 1 2 2 2
  spline S72 degree 2 poles (549.7484, 449.7048) (552.3189, 448.6934) (560.2411, 447.8506) (565.5928, 447.8506) knots 0 0 0 1 2 2 2
  spline S73 degree 2 poles (565.5928, 447.8506) (570.9445, 447.8506) (578.8245, 448.6934) (581.4793, 449.7469) knots 0 0 0 1 2 2 2
  spline S74 degree 2 poles (581.4793, 449.7469) (584.1341, 450.8004) (586.8732, 454.4665) (586.8732, 457.3741) knots 0 0 0 1 2 2 2
  spline S75 degree 2 poles (586.8732, 457.3741) (586.8732, 460.2817) (584.1341, 464.0322) (581.395, 465.1278) knots 0 0 0 1 2 2 2
  spline S76 degree 2 poles (581.395, 465.1278) (578.7403, 466.1813) (570.6495, 466.9398) (565.5506, 466.9398) knots 0 0 0 1 2 2 2
  spline S77 degree 2 poles (565.5506, 466.9398) (560.0725, 466.9398) (552.7403, 466.2655) (549.8748, 465.1699) knots 0 0 0 1 2 2 2
  spline S78 degree 2 poles (549.8748, 465.1699) (547.1779, 464.1586) (544.2702, 460.4082) (544.2702, 457.3741) knots 0 0 0 1 2 2 2
  spline S79 degree 2 poles (544.2702, 457.3741) (544.2702, 454.5087) (547.0093, 450.7582) (549.7484, 449.7048) knots 0 0 0 1 2 2 2
  line L61 (539.5928, 359.99) -> (539.5928, 385.3579)
  line L62 (539.5928, 385.3579) -> (544.9023, 385.3579)
  line L63 (544.9023, 385.3579) -> (544.9023, 375.9187)
  line L64 (544.9023, 375.9187) -> (579.7516, 375.9187)
  line L65 (579.7516, 375.9187) -> (579.7516, 385.3579)
  line L66 (579.7516, 385.3579) -> (584.5134, 385.3579)
  spline S80 degree 2 poles (584.5134, 385.3579) (584.5134, 380.0062) (587.5474, 374.9495) (591.7613, 374.6124) knots 0 0 0 1 2 2 2
  line L67 (591.7613, 374.6124) -> (591.7613, 369.2185)
  line L68 (591.7613, 369.2185) -> (544.9023, 369.2185)
  line L69 (544.9023, 369.2185) -> (544.9023, 359.99)
  line L70 (544.9023, 359.99) -> (539.5928, 359.99)
  spline S81 degree 2 poles (565.5928, 318.0613) (551.6025, 318.0613) (538.4971, 326.1942) (538.4971, 334.6642) knots 0 0 0 1 2 2 2
  spline S82 degree 2 poles (538.4971, 334.6642) (538.4971, 343.2607) (551.8553, 351.3093) (565.5506, 351.3093) knots 0 0 0 1 2 2 2
  spline S83 degree 2 poles (565.5506, 351.3093) (579.6252, 351.3093) (592.6463, 343.1764) (592.6463, 334.6642) knots 0 0 0 1 2 2 2
  spline S84 degree 2 poles (592.6463, 334.6642) (592.6463, 326.11) (579.1617, 318.0613) (565.5928, 318.0613) knots 0 0 0 1 2 2 2
  spline S85 degree 2 poles (549.7484, 326.9949) (552.3189, 325.9835) (560.2411, 325.1407) (565.5928, 325.1407) knots 0 0 0 1 2 2 2
  spline S86 degree 2 poles (565.5928, 325.1407) (570.9445, 325.1407) (578.8245, 325.9835) (581.4793, 327.037) knots 0 0 0 1 2 2 2
  spline S87 degree 2 poles (581.4793, 327.037) (584.1341, 328.0905) (586.8732, 331.7566) (586.8732, 334.6642) knots 0 0 0 1 2 2 2
  spline S88 degree 2 poles (586.8732, 334.6642) (586.8732, 337.5719) (584.1341, 341.3223) (581.395, 342.4179) knots 0 0 0 1 2 2 2
  spline S89 degree 2 poles (581.395, 342.4179) (578.7403, 343.4714) (570.6495, 344.2299) (565.5506, 344.2299) knots 0 0 0 1 2 2 2
  spline S90 degree 2 poles (565.5506, 344.2299) (560.0725, 344.2299) (552.7403, 343.5557) (549.8748, 342.46) knots 0 0 0 1 2 2 2
  spline S91 degree 2 poles (549.8748, 342.46) (547.1779, 341.4487) (544.2702, 337.6983) (544.2702, 334.6642) knots 0 0 0 1 2 2 2
  spline S92 degree 2 poles (544.2702, 334.6642) (544.2702, 331.7988) (547.0093, 328.0484) (549.7484, 326.9949) knots 0 0 0 1 2 2 2
  line L71 (539.5928, 257.0014) -> (539.5928, 289.0694)
  line L72 (539.5928, 289.0694) -> (546.9672, 289.0694)
  spline S93 degree 2 poles (546.9672, 289.0694) (550.2119, 285.614) (556.2378, 279.4617) (559.4826, 276.5119) knots 0 0 0 1 2 2 2
  spline S94 degree 2 poles (559.4826, 276.5119) (566.0142, 270.5702) (573.8521, 266.2299) (578.0239, 266.2299) knots 0 0 0 1 2 2 2
  spline S95 degree 2 poles (578.0239, 266.2299) (580.2151, 266.2299) (583.502, 267.5784) (584.5555, 268.8004) knots 0 0 0 1 2 2 2
  spline S96 degree 2 poles (584.5555, 268.8004) (585.609, 270.0224) (586.6625, 273.225) (586.6625, 275.1634) knots 0 0 0 1 2 2 2
  spline S97 degree 2 poles (586.6625, 275.1634) (586.6625, 277.0176) (585.7354, 280.8101) (585.019, 282.5378) knots 0 0 0 1 2 2 2
  spline S98 degree 2 poles (585.019, 282.5378) (584.4291, 284.0127) (582.7435, 286.7518) (582.1535, 287.5946) knots 0 0 0 1 2 2 2
  line L73 (582.1535, 287.5946) -> (582.1535, 287.9738)
  line L74 (582.1535, 287.9738) -> (589.5701, 287.9738)
  spline S99 degree 2 poles (589.5701, 287.9738) (590.6236, 285.8247) (592.6884, 278.1132) (592.6884, 274.6578) knots 0 0 0 1 2 2 2
  spline S100 degree 2 poles (592.6884, 274.6578) (592.6884, 267.3677) (584.9769, 259.1505) (578.4031, 259.1505) knots 0 0 0 1 2 2 2
  spline S101 degree 2 poles (578.4031, 259.1505) (575.327, 259.1505) (570.186, 260.5832) (567.9947, 261.8474) knots 0 0 0 1 2 2 2
  spline S102 degree 2 poles (567.9947, 261.8474) (565.7192, 263.1116) (561.2524, 266.7777) (559.1033, 268.8004) knots 0 0 0 1 2 2 2
  spline S103 degree 2 poles (559.1033, 268.8004) (555.5215, 272.0873) (547.8521, 280.1359) (545.6187, 282.5378) knots 0 0 0 1 2 2 2
  line L75 (545.6187, 282.5378) -> (545.6187, 257.0014)
  line L76 (545.6187, 257.0014) -> (539.5928, 257.0014)
  spline S104 degree 2 poles (565.5928, 217.6853) (551.6025, 217.6853) (538.4971, 225.8182) (538.4971, 234.2882) knots 0 0 0 1 2 2 2
  spline S105 degree 2 poles (538.4971, 234.2882) (538.4971, 242.8847) (551.8553, 250.9333) (565.5506, 250.9333) knots 0 0 0 1 2 2 2
  spline S106 degree 2 poles (565.5506, 250.9333) (579.6252, 250.9333) (592.6463, 242.8004) (592.6463, 234.2882) knots 0 0 0 1 2 2 2
  spline S107 degree 2 poles (592.6463, 234.2882) (592.6463, 225.7339) (579.1617, 217.6853) (565.5928, 217.6853) knots 0 0 0 1 2 2 2
  spline S108 degree 2 poles (549.7484, 226.6189) (552.3189, 225.6075) (560.2411, 224.7647) (565.5928, 224.7647) knots 0 0 0 1 2 2 2
  spline S109 degree 2 poles (565.5928, 224.7647) (570.9445, 224.7647) (578.8245, 225.6075) (581.4793, 226.661) knots 0 0 0 1 2 2 2
  spline S110 degree 2 poles (581.4793, 226.661) (584.1341, 227.7145) (586.8732, 231.3806) (586.8732, 234.2882) knots 0 0 0 1 2 2 2
  spline S111 degree 2 poles (586.8732, 234.2882) (586.8732, 237.1959) (584.1341, 240.9463) (581.395, 242.0419) knots 0 0 0 1 2 2 2
  spline S112 degree 2 poles (581.395, 242.0419) (578.7403, 243.0954) (570.6495, 243.8539) (565.5506, 243.8539) knots 0 0 0 1 2 2 2
  spline S113 degree 2 poles (565.5506, 243.8539) (560.0725, 243.8539) (552.7403, 243.1796) (549.8748, 242.084) knots 0 0 0 1 2 2 2
  spline S114 degree 2 poles (549.8748, 242.084) (547.1779, 241.0727) (544.2702, 237.3223) (544.2702, 234.2882) knots 0 0 0 1 2 2 2
  spline S115 degree 2 poles (544.2702, 234.2882) (544.2702, 231.4228) (547.0093, 227.6724) (549.7484, 226.6189) knots 0 0 0 1 2 2 2
  spline S116 degree 2 poles (586.6625, 174.661) (586.6625, 176.5573) (585.7354, 180.3077) (585.019, 182.1197) knots 0 0 0 1 2 2 2
  spline S117 degree 2 poles (585.019, 182.1197) (584.3027, 183.8053) (582.7856, 186.2915) (582.1114, 187.2607) knots 0 0 0 1 2 2 2
  line L77 (582.1114, 187.2607) -> (582.1114, 187.6821)
  line L78 (582.1114, 187.6821) -> (589.4858, 187.6821)
  spline S118 degree 2 poles (589.4858, 187.6821) (590.7078, 185.4066) (592.6884, 177.6108) (592.6884, 174.1132) knots 0 0 0 1 2 2 2
  spline S119 degree 2 poles (592.6884, 174.1132) (592.6884, 170.5735) (591.2557, 165.3061) (589.7386, 163.157) knots 0 0 0 1 2 2 2
  spline S120 degree 2 poles (589.7386, 163.157) (588.0952, 160.8814) (583.3335, 158.5216) (580.1309, 158.5216) knots 0 0 0 1 2 2 2
  spline S121 degree 2 poles (580.1309, 158.5216) (575.8326, 158.5216) (569.3432, 164.1683) (568.5004, 168.1294) knots 0 0 0 1 2 2 2
  line L79 (568.5004, 168.1294) -> (567.9947, 168.1294)
  spline S122 degree 2 poles (567.9947, 168.1294) (567.6576, 166.486) (566.1406, 162.7356) (564.6236, 161.1343) knots 0 0 0 1 2 2 2
  spline S123 degree 2 poles (564.6236, 161.1343) (563.1487, 159.533) (558.4291, 157.5103) (555.0158, 157.5103) knots 0 0 0 1 2 2 2
  spline S124 degree 2 poles (555.0158, 157.5103) (551.5182, 157.5103) (545.5766, 159.9122) (543.301, 162.1035) knots 0 0 0 1 2 2 2
  spline S125 degree 2 poles (543.301, 162.1035) (540.9412, 164.379) (538.4971, 170.8263) (538.4971, 174.9138) knots 0 0 0 1 2 2 2
  spline S126 degree 2 poles (538.4971, 174.9138) (538.4971, 178.8328) (540.3934, 186.5022) (541.6997, 189.1148) knots 0 0 0 1 2 2 2
  line L80 (541.6997, 189.1148) -> (549.0741, 189.1148)
  line L81 (549.0741, 189.1148) -> (549.0741, 188.6091)
  spline S127 degree 2 poles (549.0741, 188.6091) (547.4728, 186.4179) (544.5231, 179.0014) (544.5231, 175.3352) knots 0 0 0 1 2 2 2
  spline S128 degree 2 poles (544.5231, 175.3352) (544.5231, 173.1861) (545.8715, 168.8879) (547.4307, 167.4552) knots 0 0 0 1 2 2 2
  spline S129 degree 2 poles (547.4307, 167.4552) (548.9899, 166.0646) (552.6981, 164.5897) (555.5215, 164.5897) knots 0 0 0 1 2 2 2
  spline S130 degree 2 poles (555.5215, 164.5897) (558.3448, 164.5897) (562.0109, 166.2331) (563.0644, 167.708) knots 0 0 0 1 2 2 2
  spline S131 degree 2 poles (563.0644, 167.708) (564.1179, 169.1829) (564.9185, 173.1861) (564.9185, 175.5459) knots 0 0 0 1 2 2 2
  line L82 (564.9185, 175.5459) -> (564.9185, 178.4957)
  line L83 (564.9185, 178.4957) -> (570.6916, 178.4957)
  line L84 (570.6916, 178.4957) -> (570.6916, 176.178)
  spline S132 degree 2 poles (570.6916, 176.178) (570.6916, 171.5006) (575.1584, 165.601) (579.4145, 165.601) knots 0 0 0 1 2 2 2
  spline S133 degree 2 poles (579.4145, 165.601) (581.395, 165.601) (584.2184, 167.1181) (585.0612, 168.3401) knots 0 0 0 1 2 2 2
  spline S134 degree 2 poles (585.0612, 168.3401) (585.9461, 169.6464) (586.6625, 172.849) (586.6625, 174.661) knots 0 0 0 1 2 2 2
  spline S135 degree 2 poles (565.5928, 117.3093) (551.6025, 117.3093) (538.4971, 125.4422) (538.4971, 133.9122) knots 0 0 0 1 2 2 2
  spline S136 degree 2 poles (538.4971, 133.9122) (538.4971, 142.5087) (551.8553, 150.5573) (565.5506, 150.5573) knots 0 0 0 1 2 2 2
  spline S137 degree 2 poles (565.5506, 150.5573) (579.6252, 150.5573) (592.6463, 142.4244) (592.6463, 133.9122) knots 0 0 0 1 2 2 2
  spline S138 degree 2 poles (592.6463, 133.9122) (592.6463, 125.3579) (579.1617, 117.3093) (565.5928, 117.3093) knots 0 0 0 1 2 2 2
  spline S139 degree 2 poles (549.7484, 126.2429) (552.3189, 125.2315) (560.2411, 124.3887) (565.5928, 124.3887) knots 0 0 0 1 2 2 2
  spline S140 degree 2 poles (565.5928, 124.3887) (570.9445, 124.3887) (578.8245, 125.2315) (581.4793, 126.285) knots 0 0 0 1 2 2 2
  spline S141 degree 2 poles (581.4793, 126.285) (584.1341, 127.3385) (586.8732, 131.0046) (586.8732, 133.9122) knots 0 0 0 1 2 2 2
  spline S142 degree 2 poles (586.8732, 133.9122) (586.8732, 136.8198) (584.1341, 140.5703) (581.395, 141.6659) knots 0 0 0 1 2 2 2
  spline S143 degree 2 poles (581.395, 141.6659) (578.7403, 142.7194) (570.6495, 143.4779) (565.5506, 143.4779) knots 0 0 0 1 2 2 2
  spline S144 degree 2 poles (565.5506, 143.4779) (560.0725, 143.4779) (552.7403, 142.8036) (549.8748, 141.708) knots 0 0 0 1 2 2 2
  spline S145 degree 2 poles (549.8748, 141.708) (547.1779, 140.6967) (544.2702, 136.9463) (544.2702, 133.9122) knots 0 0 0 1 2 2 2
  spline S146 degree 2 poles (544.2702, 133.9122) (544.2702, 131.0468) (547.0093, 127.2963) (549.7484, 126.2429) knots 0 0 0 1 2 2 2
  line L85 (557.4599, 54.8587) -> (557.4599, 61.0532)
  line L86 (557.4599, 61.0532) -> (539.5928, 61.0532)
  line L87 (539.5928, 61.0532) -> (539.5928, 67.7534)
  line L88 (539.5928, 67.7534) -> (557.4599, 67.7534)
  line L89 (557.4599, 67.7534) -> (557.4599, 90.7194)
  line L90 (557.4599, 90.7194) -> (564.7921, 90.7194)
  line L91 (564.7921, 90.7194) -> (591.5928, 67.4584)
  line L92 (591.5928, 67.4584) -> (591.5928, 61.0532)
  line L93 (591.5928, 61.0532) -> (563.0644, 61.0532)
  line L94 (563.0644, 61.0532) -> (563.0644, 54.8587)
  line L95 (563.0644, 54.8587) -> (557.4599, 54.8587)
  line L96 (563.0644, 67.7534) -> (583.3756, 67.7534)
  line L97 (583.3756, 67.7534) -> (563.0644, 85.2412)
  line L98 (563.0644, 85.2412) -> (563.0644, 67.7534)
  spline S147 degree 2 poles (565.5928, 16.9333) (551.6025, 16.9333) (538.4971, 25.0662) (538.4971, 33.5362) knots 0 0 0 1 2 2 2
  spline S148 degree 2 poles (538.4971, 33.5362) (538.4971, 42.1327) (551.8553, 50.1813) (565.5506, 50.1813) knots 0 0 0 1 2 2 2
  spline S149 degree 2 poles (565.5506, 50.1813) (579.6252, 50.1813) (592.6463, 42.0484) (592.6463, 33.5362) knots 0 0 0 1 2 2 2
  spline S150 degree 2 poles (592.6463, 33.5362) (592.6463, 24.9819) (579.1617, 16.9333) (565.5928, 16.9333) knots 0 0 0 1 2 2 2
  spline S151 degree 2 poles (549.7484, 25.8669) (552.3189, 24.8555) (560.2411, 24.0127) (565.5928, 24.0127) knots 0 0 0 1 2 2 2
  spline S152 degree 2 poles (565.5928, 24.0127) (570.9445, 24.0127) (578.8245, 24.8555) (581.4793, 25.909) knots 0 0 0 1 2 2 2
  spline S153 degree 2 poles (581.4793, 25.909) (584.1341, 26.9625) (586.8732, 30.6286) (586.8732, 33.5362) knots 0 0 0 1 2 2 2
  spline S154 degree 2 poles (586.8732, 33.5362) (586.8732, 36.4438) (584.1341, 40.1942) (581.395, 41.2899) knots 0 0 0 1 2 2 2
  spline S155 degree 2 poles (581.395, 41.2899) (578.7403, 42.3434) (570.6495, 43.1019) (565.5506, 43.1019) knots 0 0 0 1 2 2 2
  spline S156 degree 2 poles (565.5506, 43.1019) (560.0725, 43.1019) (552.7403, 42.4276) (549.8748, 41.332) knots 0 0 0 1 2 2 2
  spline S157 degree 2 poles (549.8748, 41.332) (547.1779, 40.3207) (544.2702, 36.5703) (544.2702, 33.5362) knots 0 0 0 1 2 2 2
  spline S158 degree 2 poles (544.2702, 33.5362) (544.2702, 30.6707) (547.0093, 26.9203) (549.7484, 25.8669) knots 0 0 0 1 2 2 2
  spline S159 degree 2 poles (556.1114, -43.5788) (552.361, -43.5788) (545.9558, -41.1769) (543.596, -38.9857) knots 0 0 0 1 2 2 2
  spline S160 degree 2 poles (543.596, -38.9857) (541.2362, -36.7944) (538.4971, -30.2628) (538.4971, -26.2174) knots 0 0 0 1 2 2 2
  spline S161 degree 2 poles (538.4971, -26.2174) (538.4971, -22.5092) (540.1406, -15.2612) (541.4469, -12.6064) knots 0 0 0 1 2 2 2
  line L99 (541.4469, -12.6064) -> (548.8213, -12.6064)
  line L100 (548.8213, -12.6064) -> (548.8213, -13.1121)
  spline S162 degree 2 poles (548.8213, -13.1121) (548.2313, -13.9127) (546.7143, -16.9046) (546.0401, -18.7166) knots 0 0 0 1 2 2 2
  spline S163 degree 2 poles (546.0401, -18.7166) (545.3237, -20.7814) (544.5231, -24.1947) (544.5231, -26.3438) knots 0 0 0 1 2 2 2
  spline S164 degree 2 poles (544.5231, -26.3438) (544.5231, -28.4508) (546.0401, -32.4119) (547.6835, -33.8447) knots 0 0 0 1 2 2 2
  spline S165 degree 2 poles (547.6835, -33.8447) (549.2427, -35.151) (553.3723, -36.4994) (556.1535, -36.4994) knots 0 0 0 1 2 2 2
  spline S166 degree 2 poles (556.1535, -36.4994) (558.9347, -36.4994) (562.4745, -34.9824) (563.6544, -33.5497) knots 0 0 0 1 2 2 2
  spline S167 degree 2 poles (563.6544, -33.5497) (564.9607, -32.0748) (566.0563, -27.6923) (566.0563, -25.0375) knots 0 0 0 1 2 2 2
  spline S168 degree 2 poles (566.0563, -25.0375) (566.0563, -22.172) (565.1714, -16.4832) (564.7921, -14.7555) knots 0 0 0 1 2 2 2
  line L101 (564.7921, -14.7555) -> (591.5928, -14.7555)
  line L102 (591.5928, -14.7555) -> (591.5928, -43.2839)
  line L103 (591.5928, -43.2839) -> (585.4826, -43.2839)
  line L104 (585.4826, -43.2839) -> (585.4826, -21.4557)
  line L105 (585.4826, -21.4557) -> (571.6187, -21.4557)
  spline S169 degree 2 poles (571.6187, -21.4557) (571.7873, -22.7199) (571.9137, -25.1639) (571.9137, -26.1753) knots 0 0 0 1 2 2 2
  spline S170 degree 2 poles (571.9137, -26.1753) (571.9137, -30.1785) (570.6074, -35.6988) (568.6689, -38.2271) knots 0 0 0 1 2 2 2
  spline S171 degree 2 poles (568.6689, -38.2271) (566.7305, -40.7977) (560.831, -43.5788) (556.1114, -43.5788) knots 0 0 0 1 2 2 2
  spline S172 degree 2 poles (565.5928, -83.4427) (551.6025, -83.4427) (538.4971, -75.3098) (538.4971, -66.8398) knots 0 0 0 1 2 2 2
  spline S173 degree 2 poles (538.4971, -66.8398) (538.4971, -58.2434) (551.8553, -50.1947) (565.5506, -50.1947) knots 0 0 0 1 2 2 2
  spline S174 degree 2 poles (565.5506, -50.1947) (579.6252, -50.1947) (592.6463, -58.3276) (592.6463, -66.8398) knots 0 0 0 1 2 2 2
  spline S175 degree 2 poles (592.6463, -66.8398) (592.6463, -75.3941) (579.1617, -83.4427) (565.5928, -83.4427) knots 0 0 0 1 2 2 2
  spline S176 degree 2 poles (549.7484, -74.5092) (552.3189, -75.5205) (560.2411, -76.3633) (565.5928, -76.3633) knots 0 0 0 1 2 2 2
  spline S177 degree 2 poles (565.5928, -76.3633) (570.9445, -76.3633) (578.8245, -75.5205) (581.4793, -74.467) knots 0 0 0 1 2 2 2
  spline S178 degree 2 poles (581.4793, -74.467) (584.1341, -73.4135) (586.8732, -69.7474) (586.8732, -66.8398) knots 0 0 0 1 2 2 2
  spline S179 degree 2 poles (586.8732, -66.8398) (586.8732, -63.9322) (584.1341, -60.1818) (581.395, -59.0861) knots 0 0 0 1 2 2 2
  spline S180 degree 2 poles (581.395, -59.0861) (578.7403, -58.0327) (570.6495, -57.2741) (565.5506, -57.2741) knots 0 0 0 1 2 2 2